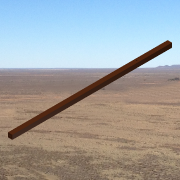
# Autodesk Inventor part: sup-stand-post
Saved by Autodesk Inventor 2013 (Build 170138000, 138)
## iProperties
Company: HERA Project
Created: 2013-06-11
Part Number: sup-stand-post
Material: Wood (Walnut)
Document SubType Name: Modeling
Designer: David DeBoer
Density: 0.55 g/cm^3
Description: Support stand post
Mass: 11457.8 g
Surface Area: 10259.2 cm^2
Volume: 20832.3 cm^3
Author: David DeBoer
Title: Support stand post
Autodesk Inventor part; units mm, degrees
ref_plane "YZ Plane" through (0, 0, 0) normal (1, 0, 0) x (0, 1, 0)
ref_plane "XZ Plane" through (0, 0, 0) normal (0, 1, 0) x (-1, 0, 0)
ref_plane "XY Plane" through (0, 0, 0) normal (0, 0, 1) x (1, 0, 0)
sketch "Sketch1" plane through (0, 0, 0) normal (0, 0, 1) x (1, 0, 0)
  line L0 (0, 0) -> (100, 0)
  line L1 (100, 0) -> (100, 100)
  line L2 (100, 100) -> (0, 100)
  line L3 (0, 100) -> (0, 0)
  dimension "d0" = 100
  dimension "d1" = 100
  constraints: 8 end point, 2 parallel, 1 horizontal, 1 perpendicular
  measures "d0" distance of L0.start L0.end
  measures "d1" distance of L2.end L0.start
extrude "Extrusion1" add sketch "Sketch1" along normal blind 3657.6
sketch "Sketch3" plane through (0, 100, 0) normal (0, 1, 0) x (1, 0, 0)
  circle A0 centre (50, -762) radius 12.7
  point P0 (0, -3657.6)
  dimension "d11" = 25.4
  dimension "d13" = 2895.6
  constraints: 1 centre point
  measures "d11" diameter of A0
  measures "d13" vertical distance of point (0, -3657.6) A0.centre
extrude "Extrusion3" cut sketch "Sketch3" against normal blind 254
sketch "Sketch4" plane through (0, 0, 3657.6) normal (0, 0, 1) x (1, 0, 0)
  circle A0 centre (50, 50) radius 12.7
  dimension "d16" = 25.4
  constraints: 1 centre point
  measures "d16" diameter of A0
extrude "Extrusion4" cut sketch "Sketch4" against normal blind 254
sketch "Sketch5" plane through (0, 0, 0) normal (0, 0, -1) x (-1, 0, 0)
  circle A0 centre (-50, 50) radius 17.9389
  constraints: 1 centre point
extrude "Extrusion5" cut sketch "Sketch5" against normal blind 25.4
body "Solid1"
